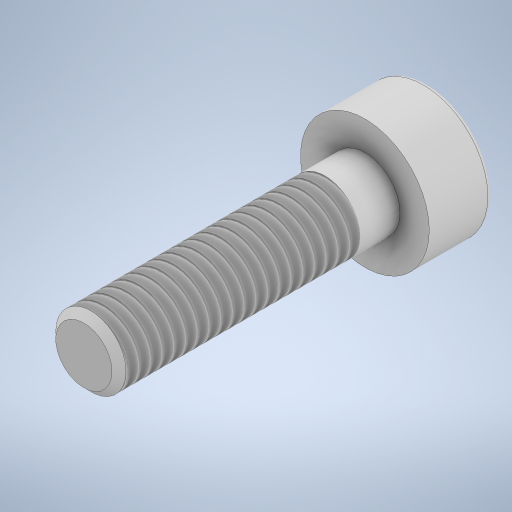
# Autodesk Inventor part: P12
Saved by Autodesk Inventor 2024 (Build 280153000, 153)
## iProperties
Created: 2023-07-07
Part Number: P12
Material: Generic
Document SubType Name: Modeling
Designer: _Astitva_Aryan_
Density: 1 g/cm^3
Appearance: Default
Author: _Astitva_Aryan_
Autodesk Inventor part; units mm, degrees
ref_plane "YZ Plane" through (0, 0, 0) normal (1, 0, 0) x (0, 1, 0)
ref_plane "XZ Plane" through (0, 0, 0) normal (0, 1, 0) x (-1, 0, 0)
ref_plane "XY Plane" through (0, 0, 0) normal (0, 0, 1) x (1, 0, 0)
sketch "Sketch1" plane through (0, 0, 0) normal (0, 0, 1) x (1, 0, 0)
  circle A0 centre (0, 0) radius 2.75
  line L0 (0, 1.4435) -> (1.2501, 0.7217)
  line L1 (1.2501, 0.7217) -> (1.2501, -0.7218)
  line L2 (1.2501, -0.7218) -> (0, -1.4435)
  line L3 (0, -1.4435) -> (-1.2501, -0.7218)
  line L4 (-1.2501, -0.7218) -> (-1.2501, 0.7217)
  line L5 (-1.2501, 0.7217) -> (0, 1.4435)
  dimension "d0" = 5.5
  dimension "d1" = 2.887
  constraints: 12 end point, 2 coincident, 1 centre point, 13 other
  measures "d0" diameter of A0
  measures "d1" distance of L2.end L0.start
extrude "Extrusion1" add sketch "Sketch1" along normal blind 2.7 contours A0 | L0 L1 L2 L3 L4 L5
extrude "Extrusion2" cut sketch "Sketch1" along normal blind 1.25 contours L0 L1 L2 L3 L4 L5
ref_plane "Work Plane1" through (0, 0, 2.7) normal (0, 0, 1) x (1, 0, 0)
sketch "Sketch2" plane through (0, 0, 2.7) normal (0, 0, 1) x (1, 0, 0)
  circle A0 centre (0, 0) radius 1.5
  dimension "d7" = 3
  constraints: 1 centre point, 1 coincident
  measures "d7" diameter of A0
extrude "Extrusion3" add sketch "Sketch2" along normal blind 12
chamfer "Chamfer1" distance 0.3 angle 45 1 edges at (-1.5, 0, 14.7)
fillet "Fillet1" radius 0.2 1 edges at (-2.75, 0, 0)
thread "Thread1" size "M3x0.5" class "6g" standard "ANSI Metric M Profile" length 10
body "Solid1"
